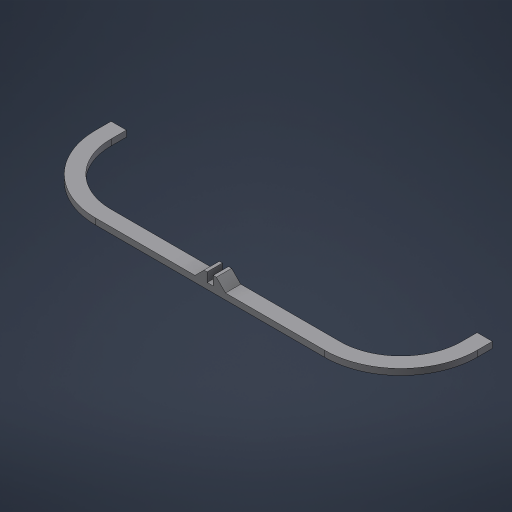
# Autodesk Inventor part: LEDholderh
Saved by Autodesk Inventor 2023.5 (Build 275446000, 446)
## iProperties
Created: 2025-03-20
Part Number: LEDholderh
Material: Generisch
Document SubType Name: Modeling
Designer: David Lill
Density: 1 g/cm^3
Appearance: Vorgabe
Author: David Lill
Autodesk Inventor part; units mm, degrees
ref_plane "YZ Plane" through (0, 0, 0) normal (1, 0, 0) x (0, 1, 0)
ref_plane "XZ Plane" through (0, 0, 0) normal (0, 1, 0) x (-1, 0, 0)
ref_plane "XY Plane" through (0, 0, 0) normal (0, 0, 1) x (1, 0, 0)
sketch "Skizze1" plane through (0, 0, 0) normal (0, 0, 1) x (1, 0, 0)
  line L0 (0, 0) -> (-37.5, 0)
  arc A0 (-62.5, 25) -> (-37.5, 0) centre (-37.5, 25) ccw
  line L1 (-62.5, 25) -> (-62.5, 30)
  line L2 (-62.5, 30) -> (-57.5, 30)
  line L3 (-57.5, 30) -> (-57.5, 25)
  arc A1 (-57.5, 25) -> (-37.5, 5) centre (-37.5, 25) ccw
  line L4 (-37.5, 5) -> (0, 5)
  line L5 (0, 5) -> (0, 0)
  line L6 (-1, 5) -> (-1, 0)
  line L7 (-5, 5) -> (-5, 0)
  point P0 (-60, 30)
  dimension "d0" = 5
  dimension "d2" = 30
  dimension "d3" = 25
  dimension "d4" = 120
  dimension "d6" = 10
  dimension "d7" = 2
  dimension "d15" = 5
  dimension "d16" = 3
  dimension "d17" = 60
  dimension "d19" = 25
  constraints: 16 end point, 6 perpendicular, 4 point on circle, 4 point on line, 4 tangent, 2 centre point, 1 concentric, 1 horizontal, 1 midpoint, 1 parallel
  measures "d0" distance of L4.end L0.start
  measures "d2" distance from line of L0.start L2
  measures "d3" radius of A0
  measures "d4" diameter of point (-60, 30) L5
  measures "d6" diameter of L7 L5
  measures "d7" diameter of L6 L5
extrude "Extrusion1" add sketch "Skizze1" along normal blind 2
extrude "Extrusion2" add sketch "Skizze1" along normal blind 5 contours L0 L7 L4 L6
mirror "Spiegeln1" about plane through (0, 0, 0) normal (1, 0, 0) of "Extrusion1", "Extrusion2"
chamfer "Fase1" distance 3 angle 45 2 edges at (-5, 2.5, 5) (5, 2.5, 5)
